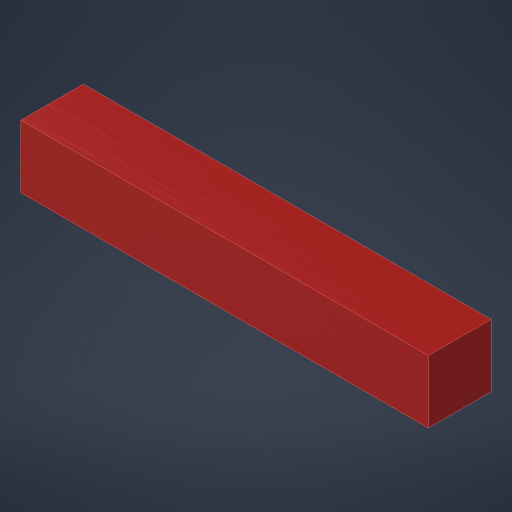
# Autodesk Inventor part: MU-005 bumper
Saved by Autodesk Inventor 2024.2 (Build 282272000, 272)
## iProperties
Created: 2025-01-05
Part Number: MU-005 bumper
Material: Generic
Document SubType Name: Modeling
Designer: brand
Density: 1 g/cm^3
Appearance: Red
Author: brand
Autodesk Inventor part; units mm, degrees
ref_plane "YZ Plane" through (0, 0, 0) normal (1, 0, 0) x (0, 1, 0)
ref_plane "XZ Plane" through (0, 0, 0) normal (0, 1, 0) x (-1, 0, 0)
ref_plane "XY Plane" through (0, 0, 0) normal (0, 0, 1) x (1, 0, 0)
sketch "Sketch1" plane through (0, 0, 0) normal (0, 0, 1) x (1, 0, 0)
  line L0 (-330.2, -50.8) -> (330.2, -50.8)
  line L1 (330.2, -50.8) -> (330.2, 50.8)
  line L2 (330.2, 50.8) -> (-330.2, 50.8)
  line L3 (-330.2, 50.8) -> (-330.2, -50.8)
  line L4 (-330.2, -50.8) -> (330.2, 50.8) construction
  line L5 (330.2, -50.8) -> (-330.2, 50.8) construction
  point P0 (0, 0)
  dimension "d0" = 101.6
  dimension "d1" = 660.4
  constraints: 12 end point, 2 midpoint, 2 parallel, 1 horizontal, 1 perpendicular
  measures "d0" distance of L2.end L0.start
  measures "d1" distance of L0.start L0.end
extrude "Extrusion1" add sketch "Sketch1" along normal mid plane 101.6
body "Solid1"
